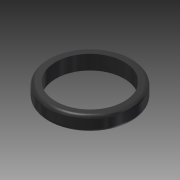
# Autodesk Inventor part: Pneu
Saved by Autodesk Inventor 2014 SP2 (Build 180246200, 246)
## iProperties
Created: 2015-03-17
Part Number: Pneu
Material: Caoutchouc
Document SubType Name: Modeling
Designer: sd
Density: 0.93 g/cm^3
Appearance: Caoutchouc - Noir - Version 1.1
Mass: 1.34121 g
Surface Area: 14.4397 cm^2
Volume: 1.44216 cm^3
Author: sd
Autodesk Inventor part; units mm, degrees
ref_plane "YZ Plane" through (0, 0, 0) normal (1, 0, 0) x (0, 1, 0)
ref_plane "XZ Plane" through (0, 0, 0) normal (0, 1, 0) x (-1, 0, 0)
ref_plane "XY Plane" through (0, 0, 0) normal (0, 0, 1) x (1, 0, 0)
sketch "Esquisse1" plane through (0, 0, 0) normal (0, 0, 1) x (1, 0, 0)
  circle A0 centre (0, 0) radius 16
  circle A1 centre (0, 0) radius 13
  dimension "d0" = 32
  dimension "d1" = 26
  constraints: 2 centre point, 2 coincident
  measures "d0" diameter of A0
  measures "d1" diameter of A1
extrude "Extrusion1" add sketch "Esquisse1" along normal blind 5.5
fillet "Congé1" radius 1.2 2 edges at (-16, 0, 5.5) (-16, 0, 0)
